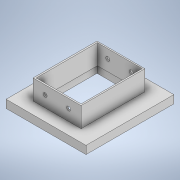
# Autodesk Inventor part: table
Saved by Autodesk Inventor 2021 (Build 250183000, 183)
## iProperties
Created: 2021-07-25
Part Number: table
Material: Generic
Document SubType Name: Modeling
Designer: aksha
Density: 1 g/cm^3
Appearance: Default
Author: aksha
Autodesk Inventor part; units mm, degrees
ref_plane "YZ Plane" through (0, 0, 0) normal (1, 0, 0) x (0, 1, 0)
ref_plane "XZ Plane" through (0, 0, 0) normal (0, 1, 0) x (-1, 0, 0)
ref_plane "XY Plane" through (0, 0, 0) normal (0, 0, 1) x (1, 0, 0)
sketch "Sketch1" plane through (0, 0, 0) normal (0, 1, 0) x (-1, 0, 0)
  line L0 (131.6438, 370.8535) -> (1131.6438, 370.8535)
  line L1 (1131.6438, 370.8535) -> (1131.6438, -729.1465)
  line L2 (1131.6438, -729.1465) -> (131.6438, -729.1465)
  line L3 (131.6438, -729.1465) -> (131.6438, 370.8535)
  point P0 (0, 0)
  dimension "d0" = 1100
  dimension "d1" = 1000
  constraints: 8 end point, 2 parallel, 1 horizontal, 1 perpendicular
  measures "d0" distance of L2.end L0.start
  measures "d1" distance of L1.end L2.end
extrude "Extrusion1" add sketch "Sketch1" along normal blind 100
sketch "Sketch2" plane through (0, 100, 0) normal (0, 1, 0) x (1, 0, 0)
  line L0 (-943.6624, -220.8535) -> (-343.6624, -220.8535)
  line L1 (-343.6624, -220.8535) -> (-343.6624, 579.1465)
  line L2 (-343.6624, 579.1465) -> (-943.6624, 579.1465)
  line L3 (-943.6624, 579.1465) -> (-943.6624, -220.8535)
  line L4 (-1131.6438, -370.8535) -> (-131.6438, -370.8535) projected
  point P0 (0, 0)
  dimension "d4" = 800
  dimension "d5" = 600
  dimension "d6" = 150
  constraints: 8 end point, 2 parallel, 1 horizontal, 1 perpendicular
  measures "d4" distance of L0.end L1.end
  measures "d5" distance of L1.end L2.end
  measures "d6" distance between parallel lines of L0 L4
extrude "Extrusion2" cut sketch "Sketch2" against normal blind 100
sketch "Sketch3" plane through (0, 100, 0) normal (0, 1, 0) x (1, 0, 0)
  line L0 (-943.6624, -220.8535) -> (-343.6624, -220.8535) projected
  line L1 (-343.6624, 579.1465) -> (-943.6624, 579.1465) projected
  line L2 (-943.6624, -220.8535) -> (-343.6624, -220.8535)
  line L3 (-343.6624, -220.8535) -> (-343.6624, 579.1465)
  line L4 (-343.6624, 579.1465) -> (-943.6624, 579.1465)
  line L5 (-943.6624, 579.1465) -> (-943.6624, -220.8535)
  line L6 (-923.4548, -202.1195) -> (-361.8828, -202.1195)
  line L7 (-361.8828, -202.1195) -> (-361.8828, 563.2076)
  line L8 (-361.8828, 563.2076) -> (-923.4548, 563.2076)
  line L9 (-923.4548, 563.2076) -> (-923.4548, -202.1195)
  point P0 (0, 0)
  point P1 (-943.6624, 579.1465)
  constraints: 16 end point, 4 parallel, 2 horizontal, 2 perpendicular
extrude "Extrusion3" add sketch "Sketch3" along normal blind 250
sketch "Sketch4" plane through (-943.6624, 100, 220.8535) normal (0, 0, 1) x (1, 0, 0)
  circle A0 centre (150.8952, 140.8463) radius 25
  circle A1 centre (444.6102, 140.8463) radius 25
  point P0 (943.6624, -100)
  dimension "d11" = 50
  dimension "d12" = 50
  constraints: 2 centre point
  measures "d11" diameter of A0
  measures "d12" diameter of A1
extrude "Extrusion4" cut sketch "Sketch4" against normal blind 2500
body "Solid1"
